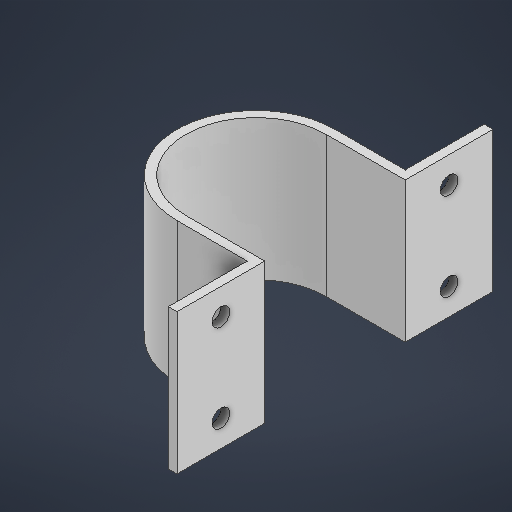
# Autodesk Inventor part: steeringbracket
Saved by Autodesk Inventor 2026.2 (Build 302298010, 298A)
## iProperties
Created: 2026-07-06
Part Number: steeringbracket
Material: Generic
Document SubType Name: Modeling
Designer: tasle
Density: 1 g/cm^3
Appearance: Default
Author: tasle
Autodesk Inventor part; units mm, degrees
ref_plane "YZ Plane" through (0, 0, 0) normal (1, 0, 0) x (0, 1, 0)
ref_plane "XZ Plane" through (0, 0, 0) normal (0, 1, 0) x (-1, 0, 0)
ref_plane "XY Plane" through (0, 0, 0) normal (0, 0, 1) x (1, 0, 0)
sketch "Sketch1" plane through (0, 0, 0) normal (0, 1, 0) x (-1, 0, 0)
  arc A0 (0, -20) -> (0, 20) centre (0, 0) ccw
  arc A1 (0, -22.5) -> (0, 22.5) centre (0, 0) ccw
  line L0 (0, 22.5) -> (-20, 22.5)
  line L1 (-22.5, 20) -> (-20, 20)
  line L2 (-20, 22.5) -> (-20, 45)
  line L3 (-20, 45) -> (-22.5, 45)
  line L4 (-22.5, 45) -> (-22.5, 20)
  line L5 (8.3208, 0) -> (-8.3208, 0)
  line L6 (0, 20) -> (-22.5, 20)
  line L7 (0, -22.5) -> (-20, -22.5)
  line L8 (-22.5, -20) -> (-20, -20)
  line L9 (-20, -22.5) -> (-20, -45)
  line L10 (-20, -45) -> (-22.5, -45)
  line L11 (-22.5, -45) -> (-22.5, -20)
  line L12 (0, -20) -> (-22.5, -20)
  point P0 (-22.5, 22.5)
  point P1 (-22.5, -22.5)
  dimension "d0" = 40
  dimension "d1" = 2.5
  dimension "d2" = 25
  constraints: 26 end point, 7 symmetric about line, 4 horizontal, 4 point on circle, 2 centre point, 2 parallel, 1 coincident, 1 midpoint, 1 perpendicular, 1 tangent
  measures "d0" diameter of A0
  measures "d1" radial gap between concentric circles of A0 A1
  measures "d2" distance of L2.end L1.end
extrude "Extrusion1" add sketch "Sketch1" along normal blind 40
sketch "Sketch2" plane through (22.5, 0, 45) normal (1, 0, 0) x (0, 0, -1)
  line L0 (12.5, 32.5) -> (77.5, 32.5)
  line L1 (77.5, 32.5) -> (77.5, 7.5)
  line L2 (77.5, 7.5) -> (12.5, 7.5)
  line L3 (12.5, 7.5) -> (12.5, 32.5)
  line L4 (0, 0) -> (0, 40) projected
  line L5 (25, 40) -> (65, 40) projected
  circle A0 centre (12.5, 32.5) radius 2.5
  circle A1 centre (77.5, 32.5) radius 2.5
  circle A2 centre (77.5, 7.5) radius 2.5
  circle A3 centre (12.5, 7.5) radius 2.5
  point P0 (45, 0)
  dimension "d5" = 65
  dimension "d6" = 25
  dimension "d7" = 12.5
  dimension "d8" = 7.5
  dimension "d9" = 5
  dimension "d10" = 5
  dimension "d11" = 5
  dimension "d12" = 5
  constraints: 8 end point, 4 centre point, 4 coincident, 2 parallel, 1 horizontal, 1 perpendicular
  measures "d5" distance of L1.end L2.end
  measures "d6" distance of L0.end L1.end
  measures "d7" distance between parallel lines of L4 L3
  measures "d8" distance between parallel lines of L5 L0
  measures "d9" diameter of A0
  measures "d10" diameter of A1
  measures "d11" diameter of A2
  measures "d12" diameter of A3
extrude "Extrusion2" cut sketch "Sketch2" against normal blind 40 contours L3 A0 L0 | L0 A0 L3 | A1 L1 L0 | L0 L1 A1 | A3 L2 L3 | L3 L2 A3 | A2 L2 L1 | L1 L2 A2
body "Solid1"
